Autodesk Inventor part; units mm, degrees
(part 2 of 2)
  spline S228 degree 2 poles (33.0997, 25.6039) (33.1113, 25.3645) (33.1113, 25.1808) knots 0 0 0 1 1 1
  line L409 (33.1113, 25.1808) -> (33.1113, 24.2835)
  line L410 (33.1113, 24.2835) -> (32.8068, 24.2835)
  line L411 (32.8068, 24.2835) -> (32.8068, 26.0875)
  line L412 (32.8068, 26.0875) -> (33.0555, 26.0875)
  line L413 (33.0555, 26.0875) -> (34.4573, 24.8902)
  line L414 (34.4573, 24.8902) -> (34.713, 24.6624)
  spline S229 degree 2 poles (34.713, 24.6624) (34.6944, 24.9135) (34.6944, 25.1343) knots 0 0 0 1 1 1
  line L415 (34.6944, 25.1343) -> (34.6944, 26.1549)
  line L416 (34.6944, 26.1549) -> (35.0176, 26.1549)
  line L417 (35.0176, 26.1549) -> (35.0176, 24.1998)
  line L418 (35.8661, 26.5129) -> (35.5151, 26.471)
  spline S230 degree 2 poles (35.5151, 26.471) (35.5476, 26.5942) (35.5476, 26.6849) knots 0 0 0 1 1 1
  spline S231 degree 2 poles (35.5476, 26.6849) (35.5476, 26.8104) (35.4639, 26.9592) (35.3895, 27.008) knots 0 0 0 1 2 2 2
  spline S232 degree 2 poles (35.3895, 27.008) (35.3337, 27.0429) (35.1106, 27.122) knots 0 0 0 1 1 1
  spline S233 degree 2 poles (35.1106, 27.122) (35.0803, 27.1313) (35.0199, 27.1545) knots 0 0 0 1 1 1
  line L419 (35.0199, 27.1545) -> (32.8068, 26.3153)
  line L420 (32.8068, 26.3153) -> (32.8068, 26.7198)
  line L421 (32.8068, 26.7198) -> (34.083, 27.1777)
  spline S234 degree 2 poles (34.083, 27.1777) (34.3248, 27.2684) (34.5922, 27.3382) knots 0 0 0 1 1 1
  spline S235 degree 2 poles (34.5922, 27.3382) (34.3411, 27.4032) (34.0947, 27.4939) knots 0 0 0 1 1 1
  line L422 (34.0947, 27.4939) -> (32.8068, 27.9658)
  line L423 (32.8068, 27.9658) -> (32.8068, 28.3401)
  line L424 (32.8068, 28.3401) -> (35.0571, 27.5009)
  spline S236 degree 2 poles (35.0571, 27.5009) (35.4197, 27.366) (35.5569, 27.2917) knots 0 0 0 1 1 1
  spline S237 degree 2 poles (35.5569, 27.2917) (35.7406, 27.1917) (35.9126, 26.9337) (35.9126, 26.7547) knots 0 0 0 1 2 2 2
  spline S238 degree 2 poles (35.9126, 26.7547) (35.9126, 26.6454) (35.8661, 26.5129) knots 0 0 0 1 1 1
  line L425 (39.573, 13.5863) -> (39.9334, 13.5863)
  line L426 (39.9334, 13.5863) -> (39.9334, 11.5708)
  spline S239 degree 2 poles (39.9334, 11.5708) (39.7985, 11.5661) (39.673, 11.615) knots 0 0 0 1 1 1
  spline S240 degree 2 poles (39.673, 11.615) (39.4661, 11.6917) (39.0686, 12.0311) (38.8059, 12.3519) knots 0 0 0 1 2 2 2
  spline S241 degree 2 poles (38.8059, 12.3519) (38.3967, 12.8471) (37.9225, 13.1958) (37.7086, 13.1958) knots 0 0 0 1 2 2 2
  spline S242 degree 2 poles (37.7086, 13.1958) (37.4855, 13.1958) (37.1809, 12.8773) (37.1809, 12.6216) knots 0 0 0 1 2 2 2
  spline S243 degree 2 poles (37.1809, 12.6216) (37.1809, 12.3519) (37.5064, 12.0288) (37.7923, 12.0264) knots 0 0 0 1 2 2 2
  line L427 (37.7923, 12.0264) -> (37.7528, 11.6405)
  spline S244 degree 2 poles (37.7528, 11.6405) (37.3227, 11.6801) (36.8717, 12.1961) (36.8717, 12.6309) knots 0 0 0 1 2 2 2
  spline S245 degree 2 poles (36.8717, 12.6309) (36.8717, 13.0702) (37.3576, 13.5817) (37.7179, 13.5817) knots 0 0 0 1 2 2 2
  spline S246 degree 2 poles (37.7179, 13.5817) (37.9016, 13.5817) (38.2549, 13.4329) (38.6455, 13.0842) (38.9872, 12.682) knots 0 0 0 1 2 3 3 3
  spline S247 degree 2 poles (38.9872, 12.682) (39.2685, 12.3449) (39.4708, 12.1543) (39.573, 12.0915) knots 0 0 0 1 2 2 2
  line L428 (39.573, 12.0915) -> (39.573, 13.5863)
  line L429 (37.2832, 14.014) -> (36.9229, 14.014)
  line L430 (36.9229, 14.014) -> (36.9229, 15.9877)
  line L431 (36.9229, 15.9877) -> (37.2135, 15.9877)
  spline S248 degree 2 poles (37.2135, 15.9877) (37.525, 15.6971) (38.5525, 15.1253) (39.0942, 14.9695) knots 0 0 0 1 2 2 2
  spline S249 degree 2 poles (39.0942, 14.9695) (39.4777, 14.8556) (39.9334, 14.8254) knots 0 0 0 1 1 1
  line L432 (39.9334, 14.8254) -> (39.9334, 14.4395)
  spline S250 degree 2 poles (39.9334, 14.4395) (39.573, 14.4464) (38.5548, 14.7161) (37.6087, 15.2206) (37.2832, 15.5065) knots 0 0 0 1 2 3 3 3
  line L433 (37.2832, 15.5065) -> (37.2832, 14.014)
  line L434 (39.573, 18.324) -> (39.9334, 18.324)
  line L435 (39.9334, 18.324) -> (39.9334, 16.3085)
  spline S251 degree 2 poles (39.9334, 16.3085) (39.7985, 16.3039) (39.673, 16.3527) knots 0 0 0 1 1 1
  spline S252 degree 2 poles (39.673, 16.3527) (39.4661, 16.4294) (39.0686, 16.7688) (38.8059, 17.0896) knots 0 0 0 1 2 2 2
  spline S253 degree 2 poles (38.8059, 17.0896) (38.3967, 17.5848) (37.9225, 17.9335) (37.7086, 17.9335) knots 0 0 0 1 2 2 2
  spline S254 degree 2 poles (37.7086, 17.9335) (37.4855, 17.9335) (37.1809, 17.615) (37.1809, 17.3593) knots 0 0 0 1 2 2 2
  spline S255 degree 2 poles (37.1809, 17.3593) (37.1809, 17.0896) (37.5064, 16.7665) (37.7923, 16.7642) knots 0 0 0 1 2 2 2
  line L436 (37.7923, 16.7642) -> (37.7528, 16.3783)
  spline S256 degree 2 poles (37.7528, 16.3783) (37.3227, 16.4178) (36.8717, 16.9339) (36.8717, 17.3686) knots 0 0 0 1 2 2 2
  spline S257 degree 2 poles (36.8717, 17.3686) (36.8717, 17.808) (37.3576, 18.3194) (37.7179, 18.3194) knots 0 0 0 1 2 2 2
  spline S258 degree 2 poles (37.7179, 18.3194) (37.9016, 18.3194) (38.2549, 18.1706) (38.6455, 17.8219) (38.9872, 17.4197) knots 0 0 0 1 2 3 3 3
  spline S259 degree 2 poles (38.9872, 17.4197) (39.2685, 17.0826) (39.4708, 16.892) (39.573, 16.8293) knots 0 0 0 1 2 2 2
  line L437 (39.573, 16.8293) -> (39.573, 18.324)
  line L438 (37.6319, 20.672) -> (37.6621, 20.3)
  spline S260 degree 2 poles (37.6621, 20.3) (37.4413, 20.2489) (37.339, 20.1582) knots 0 0 0 1 1 1
  spline S261 degree 2 poles (37.339, 20.1582) (37.1786, 20.0048) (37.1786, 19.7816) knots 0 0 0 1 1 1
  spline S262 degree 2 poles (37.1786, 19.7816) (37.1786, 19.6026) (37.2786, 19.4678) knots 0 0 0 1 1 1
  spline S263 degree 2 poles (37.2786, 19.4678) (37.4064, 19.2911) (37.9039, 19.0865) (38.3619, 19.0819) knots 0 0 0 1 2 2 2
  spline S264 degree 2 poles (38.3619, 19.0819) (38.155, 19.2167) (37.9551, 19.6096) (37.9551, 19.8235) knots 0 0 0 1 2 2 2
  spline S265 degree 2 poles (37.9551, 19.8235) (37.9551, 20.1977) (38.506, 20.7254) (38.943, 20.7254) knots 0 0 0 1 2 2 2
  spline S266 degree 2 poles (38.943, 20.7254) (39.229, 20.7254) (39.7218, 20.4767) (39.9845, 20.0443) (39.9845, 19.77) knots 0 0 0 1 2 3 3 3
  spline S267 degree 2 poles (39.9845, 19.77) (39.9845, 19.3004) (39.2964, 18.7099) (38.506, 18.7099) knots 0 0 0 1 2 2 2
  spline S268 degree 2 poles (38.506, 18.7099) (37.6226, 18.7099) (37.2204, 19.0377) knots 0 0 0 1 1 1
  spline S269 degree 2 poles (37.2204, 19.0377) (36.8717, 19.3213) (36.8717, 19.8049) knots 0 0 0 1 1 1
  spline S270 degree 2 poles (36.8717, 19.8049) (36.8717, 20.1652) (37.2762, 20.6255) (37.6319, 20.672) knots 0 0 0 1 2 2 2
  spline S271 degree 2 poles (38.9454, 19.14) (39.1383, 19.14) (39.4917, 19.3051) (39.6776, 19.598) (39.6776, 19.7607) knots 0 0 0 1 2 3 3 3
  spline S272 degree 2 poles (39.6776, 19.7607) (39.6776, 20.0001) (39.2941, 20.3395) (38.9663, 20.3395) knots 0 0 0 1 2 2 2
  spline S273 degree 2 poles (38.9663, 20.3395) (38.6501, 20.3395) (38.2852, 20.0048) (38.2852, 19.7467) knots 0 0 0 1 2 2 2
  spline S274 degree 2 poles (38.2852, 19.7467) (38.2852, 19.4934) (38.6501, 19.14) (38.9454, 19.14) knots 0 0 0 1 2 2 2
  line L439 (39.9334, 22.2946) -> (39.2034, 22.2946)
  line L440 (39.2034, 22.2946) -> (39.2034, 20.9719)
  line L441 (39.2034, 20.9719) -> (38.8594, 20.9719)
  line L442 (38.8594, 20.9719) -> (36.8834, 22.362)
  line L443 (36.8834, 22.362) -> (36.8834, 22.6689)
  line L444 (36.8834, 22.6689) -> (38.8594, 22.6689)
  line L445 (38.8594, 22.6689) -> (38.8594, 23.0804)
  line L446 (38.8594, 23.0804) -> (39.2034, 23.0804)
  line L447 (39.2034, 23.0804) -> (39.2034, 22.6689)
  line L448 (39.2034, 22.6689) -> (39.9334, 22.6689)
  line L449 (39.9334, 22.6689) -> (39.9334, 22.2946)
  line L450 (38.8594, 22.2946) -> (37.4831, 22.2946)
  line L451 (37.4831, 22.2946) -> (38.8594, 21.3392)
  line L452 (38.8594, 21.3392) -> (38.8594, 22.2946)
  spline S275 degree 2 poles (38.2782, 24.0428) (38.1922, 23.808) (37.876, 23.5825) (37.6575, 23.5825) knots 0 0 0 1 2 2 2
  spline S276 degree 2 poles (37.6575, 23.5825) (37.3251, 23.5825) (36.8717, 24.0614) (36.8717, 24.4566) knots 0 0 0 1 2 2 2
  spline S277 degree 2 poles (36.8717, 24.4566) (36.8717, 24.8564) (37.3344, 25.3423) (37.6668, 25.3423) knots 0 0 0 1 2 2 2
  spline S278 degree 2 poles (37.6668, 25.3423) (37.8783, 25.3423) (38.1922, 25.1191) (38.2782, 24.8913) knots 0 0 0 1 2 2 2
  spline S279 degree 2 poles (38.2782, 24.8913) (38.3688, 25.1749) (38.778, 25.4678) (39.0616, 25.4678) knots 0 0 0 1 2 2 2
  spline S280 degree 2 poles (39.0616, 25.4678) (39.4522, 25.4678) (39.9845, 24.9145) (39.9845, 24.4636) knots 0 0 0 1 2 2 2
  spline S281 degree 2 poles (39.9845, 24.4636) (39.9845, 24.0126) (39.4498, 23.4593) (39.05, 23.4593) knots 0 0 0 1 2 2 2
  spline S282 degree 2 poles (39.05, 23.4593) (38.7524, 23.4593) (38.3502, 23.7615) (38.2782, 24.0428) knots 0 0 0 1 2 2 2
  spline S283 degree 2 poles (39.0523, 23.8452) (39.2127, 23.8452) (39.5126, 23.9963) (39.6776, 24.2939) (39.6776, 24.4659) knots 0 0 0 1 2 3 3 3
  spline S284 degree 2 poles (39.6776, 24.4659) (39.6776, 24.7355) (39.3313, 25.0819) (39.0663, 25.0819) knots 0 0 0 1 2 2 2
  spline S285 degree 2 poles (39.0663, 25.0819) (38.7943, 25.0819) (38.4409, 24.7239) (38.4409, 24.4543) knots 0 0 0 1 2 2 2
  spline S286 degree 2 poles (38.4409, 24.4543) (38.4409, 24.1892) (38.7896, 23.8452) (39.0523, 23.8452) knots 0 0 0 1 2 2 2
  spline S287 degree 2 poles (37.6435, 23.9684) (37.8597, 23.9684) (38.1341, 24.245) (38.1341, 24.4659) knots 0 0 0 1 2 2 2
  spline S288 degree 2 poles (38.1341, 24.4659) (38.1341, 24.6821) (37.8621, 24.9564) (37.6645, 24.9564) knots 0 0 0 1 2 2 2
  spline S289 degree 2 poles (37.6645, 24.9564) (37.4599, 24.9564) (37.1786, 24.6751) (37.1786, 24.4636) knots 0 0 0 1 2 2 2
  spline S290 degree 2 poles (37.1786, 24.4636) (37.1786, 24.2474) (37.4529, 23.9684) (37.6435, 23.9684) knots 0 0 0 1 2 2 2
  line L453 (39.6752, -2.8631) -> (40.0355, -2.8631)
  line L454 (40.0355, -2.8631) -> (40.0355, -4.8786)
  spline S291 degree 2 poles (40.0355, -4.8786) (39.9007, -4.8833) (39.7752, -4.8344) knots 0 0 0 1 1 1
  spline S292 degree 2 poles (39.7752, -4.8344) (39.5683, -4.7577) (39.1707, -4.4183) (38.9081, -4.0975) knots 0 0 0 1 2 2 2
  spline S293 degree 2 poles (38.9081, -4.0975) (38.4989, -3.6024) (38.0247, -3.2537) (37.8108, -3.2537) knots 0 0 0 1 2 2 2
  spline S294 degree 2 poles (37.8108, -3.2537) (37.5876, -3.2537) (37.2831, -3.5721) (37.2831, -3.8279) knots 0 0 0 1 2 2 2
  spline S295 degree 2 poles (37.2831, -3.8279) (37.2831, -4.0975) (37.6086, -4.4206) (37.8945, -4.423) knots 0 0 0 1 2 2 2
  line L455 (37.8945, -4.423) -> (37.855, -4.8089)
  spline S296 degree 2 poles (37.855, -4.8089) (37.4249, -4.7694) (36.9739, -4.2533) (36.9739, -3.8186) knots 0 0 0 1 2 2 2
  spline S297 degree 2 poles (36.9739, -3.8186) (36.9739, -3.3792) (37.4598, -2.8678) (37.8201, -2.8678) knots 0 0 0 1 2 2 2
  spline S298 degree 2 poles (37.8201, -2.8678) (38.0038, -2.8678) (38.3571, -3.0165) (38.7477, -3.3652) (39.0894, -3.7674) knots 0 0 0 1 2 3 3 3
  spline S299 degree 2 poles (39.0894, -3.7674) (39.3707, -4.1045) (39.5729, -4.2951) (39.6752, -4.3579) knots 0 0 0 1 2 2 2
  line L456 (39.6752, -4.3579) -> (39.6752, -2.8631)
  line L457 (37.3854, -2.4354) -> (37.0251, -2.4354)
  line L458 (37.0251, -2.4354) -> (37.0251, -0.4617)
  line L459 (37.0251, -0.4617) -> (37.3156, -0.4617)
  spline S300 degree 2 poles (37.3156, -0.4617) (37.6272, -0.7523) (38.6547, -1.3242) (39.1963, -1.4799) knots 0 0 0 1 2 2 2
  spline S301 degree 2 poles (39.1963, -1.4799) (39.5799, -1.5938) (40.0355, -1.624) knots 0 0 0 1 1 1
  line L460 (40.0355, -1.624) -> (40.0355, -2.0099)
  spline S302 degree 2 poles (40.0355, -2.0099) (39.6752, -2.003) (38.657, -1.7333) (37.7108, -1.2288) (37.3854, -0.9429) knots 0 0 0 1 2 3 3 3
  line L461 (37.3854, -0.9429) -> (37.3854, -2.4354)
  line L462 (39.6752, 1.8746) -> (40.0355, 1.8746)
  line L463 (40.0355, 1.8746) -> (40.0355, -0.1409)
  spline S303 degree 2 poles (40.0355, -0.1409) (39.9007, -0.1455) (39.7752, -0.0967) knots 0 0 0 1 1 1
  spline S304 degree 2 poles (39.7752, -0.0967) (39.5683, -0.02) (39.1707, 0.3194) (38.9081, 0.6402) knots 0 0 0 1 2 2 2
  spline S305 degree 2 poles (38.9081, 0.6402) (38.4989, 1.1354) (38.0247, 1.4841) (37.8108, 1.4841) knots 0 0 0 1 2 2 2
  spline S306 degree 2 poles (37.8108, 1.4841) (37.5876, 1.4841) (37.2831, 1.1656) (37.2831, 0.9099) knots 0 0 0 1 2 2 2
  spline S307 degree 2 poles (37.2831, 0.9099) (37.2831, 0.6402) (37.6086, 0.3171) (37.8945, 0.3148) knots 0 0 0 1 2 2 2
  line L464 (37.8945, 0.3148) -> (37.855, -0.0711)
  spline S308 degree 2 poles (37.855, -0.0711) (37.4249, -0.0316) (36.9739, 0.4845) (36.9739, 0.9192) knots 0 0 0 1 2 2 2
  spline S309 degree 2 poles (36.9739, 0.9192) (36.9739, 1.3585) (37.4598, 1.87) (37.8201, 1.87) knots 0 0 0 1 2 2 2
  spline S310 degree 2 poles (37.8201, 1.87) (38.0038, 1.87) (38.3571, 1.7212) (38.7477, 1.3725) (39.0894, 0.9703) knots 0 0 0 1 2 3 3 3
  spline S311 degree 2 poles (39.0894, 0.9703) (39.3707, 0.6332) (39.5729, 0.4426) (39.6752, 0.3798) knots 0 0 0 1 2 2 2
  line L465 (39.6752, 0.3798) -> (39.6752, 1.8746)
  line L466 (37.3854, 2.3024) -> (37.0251, 2.3024)
  line L467 (37.0251, 2.3024) -> (37.0251, 4.276)
  line L468 (37.0251, 4.276) -> (37.3156, 4.276)
  spline S312 degree 2 poles (37.3156, 4.276) (37.6272, 3.9854) (38.6547, 3.4136) (39.1963, 3.2578) knots 0 0 0 1 2 2 2
  spline S313 degree 2 poles (39.1963, 3.2578) (39.5799, 3.1439) (40.0355, 3.1137) knots 0 0 0 1 1 1
  line L469 (40.0355, 3.1137) -> (40.0355, 2.7278)
  spline S314 degree 2 poles (40.0355, 2.7278) (39.6752, 2.7348) (38.657, 3.0044) (37.7108, 3.5089) (37.3854, 3.7948) knots 0 0 0 1 2 3 3 3
  line L470 (37.3854, 3.7948) -> (37.3854, 2.3024)
  line L471 (39.6752, 6.6124) -> (40.0355, 6.6124)
  line L472 (40.0355, 6.6124) -> (40.0355, 4.5968)
  spline S315 degree 2 poles (40.0355, 4.5968) (39.9007, 4.5922) (39.7752, 4.641) knots 0 0 0 1 1 1
  spline S316 degree 2 poles (39.7752, 4.641) (39.5683, 4.7177) (39.1707, 5.0571) (38.9081, 5.3779) knots 0 0 0 1 2 2 2
  spline S317 degree 2 poles (38.9081, 5.3779) (38.4989, 5.8731) (38.0247, 6.2218) (37.8108, 6.2218) knots 0 0 0 1 2 2 2
  spline S318 degree 2 poles (37.8108, 6.2218) (37.5876, 6.2218) (37.2831, 5.9033) (37.2831, 5.6476) knots 0 0 0 1 2 2 2
  spline S319 degree 2 poles (37.2831, 5.6476) (37.2831, 5.3779) (37.6086, 5.0548) (37.8945, 5.0525) knots 0 0 0 1 2 2 2
  line L473 (37.8945, 5.0525) -> (37.855, 4.6666)
  spline S320 degree 2 poles (37.855, 4.6666) (37.4249, 4.7061) (36.9739, 5.2222) (36.9739, 5.6569) knots 0 0 0 1 2 2 2
  spline S321 degree 2 poles (36.9739, 5.6569) (36.9739, 6.0963) (37.4598, 6.6077) (37.8201, 6.6077) knots 0 0 0 1 2 2 2
  spline S322 degree 2 poles (37.8201, 6.6077) (38.0038, 6.6077) (38.3571, 6.4589) (38.7477, 6.1102) (39.0894, 5.708) knots 0 0 0 1 2 3 3 3
  spline S323 degree 2 poles (39.0894, 5.708) (39.3707, 5.371) (39.5729, 5.1803) (39.6752, 5.1176) knots 0 0 0 1 2 2 2
  line L474 (39.6752, 5.1176) -> (39.6752, 6.6124)
  line L475 (39.3288, 7.0703) -> (39.2963, 7.4306)
  spline S324 degree 2 poles (39.2963, 7.4306) (39.5497, 7.4771) (39.7798, 7.7352) (39.7798, 7.9351) knots 0 0 0 1 2 2 2
  spline S325 degree 2 poles (39.7798, 7.9351) (39.7798, 8.1071) (39.6217, 8.3698) (39.3567, 8.5349) (38.9081, 8.6465) (38.6733, 8.6465) knots 0 0 0 1 2 3 4 4 4
  spline S326 degree 2 poles (38.6733, 8.6465) (38.65, 8.6465) (38.5989, 8.6441) knots 0 0 0 1 1 1
  spline S327 degree 2 poles (38.5989, 8.6441) (38.7779, 8.5326) (39.001, 8.1443) (39.001, 7.9165) knots 0 0 0 1 2 2 2
  spline S328 degree 2 poles (39.001, 7.9165) (39.001, 7.5376) (38.4524, 7.0145) (38.0038, 7.0145) knots 0 0 0 1 2 2 2
  spline S329 degree 2 poles (38.0038, 7.0145) (37.5388, 7.0145) (36.9739, 7.5608) (36.9739, 7.9723) knots 0 0 0 1 2 2 2
  spline S330 degree 2 poles (36.9739, 7.9723) (36.9739, 8.2699) (37.2947, 8.7627) (37.8875, 9.0184) (38.4478, 9.0184) knots 0 0 0 1 2 3 3 3
  spline S331 degree 2 poles (38.4478, 9.0184) (39.0336, 9.0184) (39.724, 8.765) (40.0867, 8.2629) (40.0867, 7.9258) knots 0 0 0 1 2 3 3 3
  spline S332 degree 2 poles (40.0867, 7.9258) (40.0867, 7.5701) (39.6892, 7.1168) (39.3288, 7.0703) knots 0 0 0 1 2 2 2
  spline S333 degree 2 poles (37.9852, 8.6023) (37.662, 8.6023) (37.2831, 8.2606) (37.2831, 8.0188) knots 0 0 0 1 2 2 2
  spline S334 degree 2 poles (37.2831, 8.0188) (37.2831, 7.7677) (37.6899, 7.4004) (38.0154, 7.4004) knots 0 0 0 1 2 2 2
  spline S335 degree 2 poles (38.0154, 7.4004) (38.306, 7.4004) (38.6709, 7.7491) (38.6709, 8.0095) knots 0 0 0 1 2 2 2
  spline S336 degree 2 poles (38.6709, 8.0095) (38.6709, 8.2675) (38.306, 8.6023) (37.9852, 8.6023) knots 0 0 0 1 2 2 2
  line L476 (39.6752, -19.4476) -> (40.0355, -19.4476)
  line L477 (40.0355, -19.4476) -> (40.0355, -21.4631)
  spline S337 degree 2 poles (40.0355, -21.4631) (39.9007, -21.4678) (39.7752, -21.419) knots 0 0 0 1 1 1
  spline S338 degree 2 poles (39.7752, -21.419) (39.5683, -21.3423) (39.1707, -21.0029) (38.9081, -20.682) knots 0 0 0 1 2 2 2
  spline S339 degree 2 poles (38.9081, -20.682) (38.4989, -20.1869) (38.0247, -19.8382) (37.8108, -19.8382) knots 0 0 0 1 2 2 2
  spline S340 degree 2 poles (37.8108, -19.8382) (37.5876, -19.8382) (37.2831, -20.1567) (37.2831, -20.4124) knots 0 0 0 1 2 2 2
  spline S341 degree 2 poles (37.2831, -20.4124) (37.2831, -20.682) (37.6086, -21.0052) (37.8945, -21.0075) knots 0 0 0 1 2 2 2
  line L478 (37.8945, -21.0075) -> (37.855, -21.3934)
  spline S342 degree 2 poles (37.855, -21.3934) (37.4249, -21.3539) (36.9739, -20.8378) (36.9739, -20.4031) knots 0 0 0 1 2 2 2
  spline S343 degree 2 poles (36.9739, -20.4031) (36.9739, -19.9637) (37.4598, -19.4523) (37.8201, -19.4523) knots 0 0 0 1 2 2 2
  spline S344 degree 2 poles (37.8201, -19.4523) (38.0038, -19.4523) (38.3571, -19.6011) (38.7477, -19.9498) (39.0894, -20.3519) knots 0 0 0 1 2 3 3 3
  spline S345 degree 2 poles (39.0894, -20.3519) (39.3707, -20.689) (39.5729, -20.8796) (39.6752, -20.9424) knots 0 0 0 1 2 2 2
  line L479 (39.6752, -20.9424) -> (39.6752, -19.4476)
  line L480 (37.3854, -19.0199) -> (37.0251, -19.0199)
  line L481 (37.0251, -19.0199) -> (37.0251, -17.0462)
  line L482 (37.0251, -17.0462) -> (37.3156, -17.0462)
  spline S346 degree 2 poles (37.3156, -17.0462) (37.6272, -17.3368) (38.6547, -17.9087) (39.1963, -18.0644) knots 0 0 0 1 2 2 2
  spline S347 degree 2 poles (39.1963, -18.0644) (39.5799, -18.1783) (40.0355, -18.2086) knots 0 0 0 1 1 1
  line L483 (40.0355, -18.2086) -> (40.0355, -18.5945)
  spline S348 degree 2 poles (40.0355, -18.5945) (39.6752, -18.5875) (38.657, -18.3178) (37.7108, -17.8134) (37.3854, -17.5274) knots 0 0 0 1 2 3 3 3
  line L484 (37.3854, -17.5274) -> (37.3854, -19.0199)
  line L485 (39.6752, -14.7099) -> (40.0355, -14.7099)
  line L486 (40.0355, -14.7099) -> (40.0355, -16.7254)
  spline S349 degree 2 poles (40.0355, -16.7254) (39.9007, -16.7301) (39.7752, -16.6812) knots 0 0 0 1 1 1
  spline S350 degree 2 poles (39.7752, -16.6812) (39.5683, -16.6045) (39.1707, -16.2651) (38.9081, -15.9443) knots 0 0 0 1 2 2 2
  spline S351 degree 2 poles (38.9081, -15.9443) (38.4989, -15.4492) (38.0247, -15.1004) (37.8108, -15.1004) knots 0 0 0 1 2 2 2
  spline S352 degree 2 poles (37.8108, -15.1004) (37.5876, -15.1004) (37.2831, -15.4189) (37.2831, -15.6746) knots 0 0 0 1 2 2 2
  spline S353 degree 2 poles (37.2831, -15.6746) (37.2831, -15.9443) (37.6086, -16.2674) (37.8945, -16.2698) knots 0 0 0 1 2 2 2
  line L487 (37.8945, -16.2698) -> (37.855, -16.6557)
  spline S354 degree 2 poles (37.855, -16.6557) (37.4249, -16.6162) (36.9739, -16.1001) (36.9739, -15.6654) knots 0 0 0 1 2 2 2
  spline S355 degree 2 poles (36.9739, -15.6654) (36.9739, -15.226) (37.4598, -14.7146) (37.8201, -14.7146) knots 0 0 0 1 2 2 2
  spline S356 degree 2 poles (37.8201, -14.7146) (38.0038, -14.7146) (38.3571, -14.8633) (38.7477, -15.212) (39.0894, -15.6142) knots 0 0 0 1 2 3 3 3
  spline S357 degree 2 poles (39.0894, -15.6142) (39.3707, -15.9513) (39.5729, -16.1419) (39.6752, -16.2047) knots 0 0 0 1 2 2 2
  line L488 (39.6752, -16.2047) -> (39.6752, -14.7099)
  line L489 (37.3854, -14.2822) -> (37.0251, -14.2822)
  line L490 (37.0251, -14.2822) -> (37.0251, -12.3085)
  line L491 (37.0251, -12.3085) -> (37.3156, -12.3085)
  spline S358 degree 2 poles (37.3156, -12.3085) (37.6272, -12.5991) (38.6547, -13.171) (39.1963, -13.3267) knots 0 0 0 1 2 2 2
  spline S359 degree 2 poles (39.1963, -13.3267) (39.5799, -13.4406) (40.0355, -13.4708) knots 0 0 0 1 1 1
  line L492 (40.0355, -13.4708) -> (40.0355, -13.8567)
  spline S360 degree 2 poles (40.0355, -13.8567) (39.6752, -13.8498) (38.657, -13.5801) (37.7108, -13.0756) (37.3854, -12.7897) knots 0 0 0 1 2 3 3 3
  line L493 (37.3854, -12.7897) -> (37.3854, -14.2822)
  line L494 (39.6752, -9.9722) -> (40.0355, -9.9722)
  line L495 (40.0355, -9.9722) -> (40.0355, -11.9877)
  spline S361 degree 2 poles (40.0355, -11.9877) (39.9007, -11.9923) (39.7752, -11.9435) knots 0 0 0 1 1 1
  spline S362 degree 2 poles (39.7752, -11.9435) (39.5683, -11.8668) (39.1707, -11.5274) (38.9081, -11.2066) knots 0 0 0 1 2 2 2
  spline S363 degree 2 poles (38.9081, -11.2066) (38.4989, -10.7114) (38.0247, -10.3627) (37.8108, -10.3627) knots 0 0 0 1 2 2 2
  spline S364 degree 2 poles (37.8108, -10.3627) (37.5876, -10.3627) (37.2831, -10.6812) (37.2831, -10.9369) knots 0 0 0 1 2 2 2
  spline S365 degree 2 poles (37.2831, -10.9369) (37.2831, -11.2066) (37.6086, -11.5297) (37.8945, -11.532) knots 0 0 0 1 2 2 2
  line L496 (37.8945, -11.532) -> (37.855, -11.9179)
  spline S366 degree 2 poles (37.855, -11.9179) (37.4249, -11.8784) (36.9739, -11.3623) (36.9739, -10.9276) knots 0 0 0 1 2 2 2
  spline S367 degree 2 poles (36.9739, -10.9276) (36.9739, -10.4883) (37.4598, -9.9768) (37.8201, -9.9768) knots 0 0 0 1 2 2 2
  spline S368 degree 2 poles (37.8201, -9.9768) (38.0038, -9.9768) (38.3571, -10.1256) (38.7477, -10.4743) (39.0894, -10.8765) knots 0 0 0 1 2 3 3 3
  spline S369 degree 2 poles (39.0894, -10.8765) (39.3707, -11.2136) (39.5729, -11.4042) (39.6752, -11.467) knots 0 0 0 1 2 2 2
  line L497 (39.6752, -11.467) -> (39.6752, -9.9722)
  line L498 (37.7341, -7.6242) -> (37.7643, -7.9962)
  spline S370 degree 2 poles (37.7643, -7.9962) (37.5435, -8.0473) (37.4412, -8.138) knots 0 0 0 1 1 1
  spline S371 degree 2 poles (37.4412, -8.138) (37.2808, -8.2914) (37.2808, -8.5146) knots 0 0 0 1 1 1
  spline S372 degree 2 poles (37.2808, -8.5146) (37.2808, -8.6936) (37.3807, -8.8284) knots 0 0 0 1 1 1
  spline S373 degree 2 poles (37.3807, -8.8284) (37.5086, -9.0051) (38.0061, -9.2097) (38.464, -9.2143) knots 0 0 0 1 2 2 2
  spline S374 degree 2 poles (38.464, -9.2143) (38.2571, -9.0795) (38.0572, -8.6866) (38.0572, -8.4727) knots 0 0 0 1 2 2 2
  spline S375 degree 2 poles (38.0572, -8.4727) (38.0572, -8.0985) (38.6082, -7.5708) (39.0452, -7.5708) knots 0 0 0 1 2 2 2
  spline S376 degree 2 poles (39.0452, -7.5708) (39.3312, -7.5708) (39.824, -7.8195) (40.0867, -8.2519) (40.0867, -8.5262) knots 0 0 0 1 2 3 3 3
  spline S377 degree 2 poles (40.0867, -8.5262) (40.0867, -8.9958) (39.3986, -9.5863) (38.6082, -9.5863) knots 0 0 0 1 2 2 2
  spline S378 degree 2 poles (38.6082, -9.5863) (37.7248, -9.5863) (37.3226, -9.2585) knots 0 0 0 1 1 1
  spline S379 degree 2 poles (37.3226, -9.2585) (36.9739, -8.9749) (36.9739, -8.4913) knots 0 0 0 1 1 1
  spline S380 degree 2 poles (36.9739, -8.4913) (36.9739, -8.131) (37.3784, -7.6707) (37.7341, -7.6242) knots 0 0 0 1 2 2 2
  spline S381 degree 2 poles (39.0475, -9.1562) (39.2405, -9.1562) (39.5938, -8.9912) (39.7798, -8.6982) (39.7798, -8.5355) knots 0 0 0 1 2 3 3 3
  spline S382 degree 2 poles (39.7798, -8.5355) (39.7798, -8.2961) (39.3962, -7.9567) (39.0685, -7.9567) knots 0 0 0 1 2 2 2
  spline S383 degree 2 poles (39.0685, -7.9567) (38.7523, -7.9567) (38.3873, -8.2914) (38.3873, -8.5495) knots 0 0 0 1 2 2 2
  spline S384 degree 2 poles (38.3873, -8.5495) (38.3873, -8.8029) (38.7523, -9.1562) (39.0475, -9.1562) knots 0 0 0 1 2 2 2
  point P0 (0, 0)
  point P1 (31.1984, -14.0793)
  point P2 (31.9676, 14.4059)
  point P3 (36.9739, -22.6819)
  point P4 (31.6611, -3.9848)
  point P5 (36.8717, 11.4429)
  point P6 (36.9739, -5.0065)
  constraints: 6 other
extrude "Wyciągnięcie proste3" cut sketch "Szkic4" against normal blind 1 contours L0 S177 S176 L2 L3 | S177 S178 L0 | L0 S178 S179 L2 L329 L330 L331 S180 S181 L332 L333 L334 S176 S177 | L0 L1 L2 S179 S178 | L2 L334 S175 S176 | L334 L333 L332 S181 S180 L331 L330 L329 L2 | S179 L328 L329 L2 | L4 S186 S185 L10 L11 | S186 L341 S187 S188 S0 L6 L5 L4 | L4 L5 L6 S0 S188 S189 S4 L342 L343 L344 L345 L346 S190 S191 S192 S193 L347 L348 L349 L350 L10 S185 S186 | L10 S4 L350 L337 L338 L339 L340 S185 | L350 L349 L348 L347 S193 S192 S191 S190 L346 L345 L344 L343 L342 S4 | S0 L363 S4 S189 S188 | S4 S189 L342 | L363 L364 L351 L352 S1 S0 | S0 S1 L352 S3 L359 L360 L361 S4 L363 | S4 S3 L361 L362 L363 | S1 S2 L7 L368 S196 S195 L8 L9 L357 L356 L355 S3 L352 | L352 L353 L354 L355 S3 L9 L357 L358 L359 | L361 L360 L359 S3 | L355 L356 L357 L9 S3 | L368 S197 S198 S199 L369 L370 L371 L372 L373 L16 L15 L14 L375 L376 L13 S6 S194 S195 L8 L7 | L7 L8 S195 S196 L368 | S194 L367 L366 L365 L20 L21 L22 L23 S7 S8 L12 S5 S6 | S6 L13 L376 L377 L378 L16 L17 L379 L19 L20 L365 L366 L367 S194 | L13 L14 L375 L374 L373 L16 L378 L377 L376 | L14 L15 L16 L373 L374 L375 | L20 L19 L379 L365 | L378 L379 L17 L16 | L379 L17 L18 L19 | L24 S9 S10 S11 S12 S13 L25 S14 S15 | L27 L28 L29 S19 S20 L30 S21 S22 S23 L31 L32 | L33 L34 L35 S24 S25 S26 L36 L37 L38 S27 S28 L39 L40 | L41 S29 S30 S31 S32 S33 L42 S34 S35 | L44 S39 S40 L45 L46 L47 L48 L49 L50 L51 L52 L53 L54 L55 S41 S42 | L56 S43 S44 S45 L57 L58 L59 S46 S47 S48 L60 L61 L62 L63 | L64 L65 L66 L67 L68 L69 L70 L71 S49 S50 L72 L73 L74 | L79 S53 S54 L80 L81 S55 S56 | L86 L87 L88 L89 L90 S61 S62 S63 L91 S64 S65 L92 L93 L94 L95 | L98 L99 L100 S70 S71 S72 L101 S73 S74 S75 L102 L103 L104 L105 L106 S76 S77 S78 L107 S79 S80 S81 L108 L109 | L110 L111 L112 L113 S82 S83 L114 S84 S85 L115 L116 L117 L118 L119 S86 L120 S87 L121 L122 L123 | L124 S88 S89 S90 S91 S92 S93 S94 S95 S96 L125 S97 S98 S99 L126 L127 S100 S101 | L129 L130 L131 L132 L133 L134 L135 L136 L137 L138 L139 L140 L141 L142 L143 L144 L145 L146 L147 L148 L149 L150 L151 L152 L153 | L154 L155 L156 S105 S106 S107 L157 S108 S109 S110 L158 L159 L160 L161 L162 L163 L164 L165 L166 L167 L168 | L169 L170 L171 L172 L173 L174 L175 L176 L177 L178 L179 L180 | L181 L182 L183 L184 L185 L186 L187 S111 S112 L188 L189 L190 L191 L192 L193 L194 L195 L196 L197 L198 S113 S114 L199 L200 L201 | L202 L203 L204 L205 S115 S116 L206 S117 S118 L207 L208 L209 L210 L211 S119 L212 S120 L213 L214 L215 | S121 S122 S123 S124 S125 L216 L217 L218 L219 S126 S127 L220 L221 L222 | L225 L226 S131 S132 S133 L227 S134 S135 S136 L228 L229 L230 L231 L232 L233 L234 L235 L236 | L237 L238 L239 L240 L241 L242 L243 S137 S138 L244 L245 L246 L247 L248 L249 L250 L251 L252 L253 L254 S139 S140 L255 L256 L257 | S141 S142 S143 S144 S145 L258 L259 L260 L261 S146 S147 L262 L263 L264 | L267 L268 L269 L270 S151 S152 L271 S153 S154 L272 L273 L274 L275 L276 S155 L277 S156 L278 L279 L280 | L281 L282 L283 L284 L285 S157 S158 L286 L287 L288 L289 L290 S159 S160 L291 L292 L293 L294 L295 | S161 S162 S163 L296 L297 S164 S165 L298 L299 L300 L301 L302 L303 L304 L305 L306 L307 S166 S167 S168 S169 L308 L309 S170 S171 L310 L311 | L314 L315 L316 L317 L318 L319 L320 L321 L322 L323 L324 L325 L326 L327 | L380 L381 S200 S201 S202 S203 L382 L383 L384 S204 S205 L385 L386 L387 | L391 L392 S208 L393 L394 L395 L396 L397 L398 S209 L399 L400 L401 | L402 S210 S211 S212 S213 S214 L403 S215 S216 | L405 S220 S221 S222 S223 L406 S224 S225 S226 S227 | L407 L408 S228 L409 L410 L411 L412 L413 L414 S229 L415 L416 L417 | L418 S230 S231 S232 S233 L419 L420 L421 S234 S235 L422 L423 L424 S236 S237 S238 | L425 L426 S239 S240 S241 S242 S243 L427 S244 S245 S246 S247 L428 | L429 L430 L431 S248 S249 L432 S250 L433 | L434 L435 S251 S252 S253 S254 S255 L436 S256 S257 S258 S259 L437 | L438 S260 S261 S262 S263 S264 S265 S266 S267 S268 S269 S270 | L439 L440 L441 L442 L443 L444 L445 L446 L447 L448 L449 | S275 S276 S277 S278 S279 S280 S281 S282 | L453 L454 S291 S292 S293 S294 S295 L455 S296 S297 S298 S299 L456 | L457 L458 L459 S300 S301 L460 S302 L461 | L462 L463 S303 S304 S305 S306 S307 L464 S308 S309 S310 S311 L465 | L466 L467 L468 S312 S313 L469 S314 L470 | L471 L472 S315 S316 S317 S318 S319 L473 S320 S321 S322 S323 L474 | L475 S324 S325 S326 S327 S328 S329 S330 S331 S332 | L476 L477 S337 S338 S339 S340 S341 L478 S342 S343 S344 S345 L479 | L480 L481 L482 S346 S347 L483 S348 L484 | L485 L486 S349 S350 S351 S352 S353 L487 S354 S355 S356 S357 L488 | L489 L490 L491 S358 S359 L492 S360 L493 | L494 L495 S361 S362 S363 S364 S365 L496 S366 S367 S368 S369 L497 | L498 S370 S371 S372 S373 S374 S375 S376 S377 S378 S379 S380
sketch "Szkic7" plane through (-96, 3, -40) normal (0, 0, 1) x (1, 0, 0)
  line L0 (0, 27) -> (120, 27) projected
  line L1 (0, 0) -> (21, 27)
  line L2 (0, 27) -> (21, 27)
  line L3 (0, 0) -> (0, 27)
  point P0 (96, -3)
  constraints: 6 end point, 1 perpendicular, 1 point on line
extrude "Wyciągnięcie proste4" cut sketch "Szkic7" along normal mid plane 200
